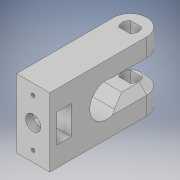
# Autodesk Inventor part: joint_2_part1
Saved by Autodesk Inventor 2019 (Build 230136000, 136)
## iProperties
Created: 2019-12-26
Part Number: joint_2_part1
Material: Типовые
Document SubType Name: Modeling
Designer: Петров Иван
Density: 1 g/cm^3
Appearance: По умолчанию
Author: Петров Иван
Autodesk Inventor part; units mm, degrees
ref_plane "YZ Plane" through (0, 0, 0) normal (1, 0, 0) x (0, 1, 0)
ref_plane "XZ Plane" through (0, 0, 0) normal (0, 1, 0) x (-1, 0, 0)
ref_plane "XY Plane" through (0, 0, 0) normal (0, 0, 1) x (1, 0, 0)
sketch "Эскиз1" plane through (0, 0, 0) normal (0, 1, 0) x (-1, 0, 0)
  arc A0 (6.0208, -6) -> (6.0208, 6) centre (0, 0) ccw
  line L0 (6.0208, -6) -> (-6.0208, -6)
  arc A1 (-6.0208, 6) -> (-6.0208, -6) centre (0, 0) ccw
  line L1 (6.0208, 6) -> (-6.0208, 6)
  line L2 (17.5, 37) -> (-17.5, 37)
  line L3 (-17.5, 37) -> (-17.5, 0)
  arc A2 (-17.5, 0) -> (17.5, 0) centre (0, 0) ccw
  line L4 (17.5, 0) -> (17.5, 37)
  line L5 (17.5, 0) -> (17.5, 57)
  line L6 (-17.5, 37) -> (17.5, 37)
  line L7 (17.5, 37) -> (17.5, 57)
  line L8 (17.5, 57) -> (-17.5, 57)
  line L9 (-17.5, 57) -> (-17.5, 37)
  constraints: 20 end point, 6 point on circle, 3 centre point, 2 parallel, 1 horizontal, 1 perpendicular
extrude "Выдавливание1" add sketch "Эскиз1" along normal blind 27
sketch "Эскиз2" plane through (-17.5, 0, 57) normal (0, 0, 1) x (1, 0, 0)
  line L0 (0, 0) -> (35, 0)
  line L1 (35, 0) -> (35, 72.2)
  line L2 (35, 72.2) -> (0, 72.2)
  line L3 (0, 72.2) -> (0, 0)
  point P0 (17.5, 0)
  dimension "d2" = 72.2
  constraints: 8 end point, 2 parallel, 1 horizontal, 1 perpendicular
  measures "d2" distance of L1.end L0.end
extrude "Выдавливание2" add sketch "Эскиз2" along normal blind 27
ref_plane "РабПлоскость1" through (17.5, 36.1, 84) normal (0, 1, 0) x (1, 0, 0)
mirror "Зеркальное отражение1" about plane through (17.5, 36.1, 84) normal (0, 1, 0) of "Выдавливание1"
sketch "Эскиз3" plane through (17.5, 0, 0) normal (1, 0, 0) x (0, 0, -1)
  line L0 (-57, 45.2) -> (-57, 27) projected
  line L1 (-57, 36.1) -> (-42, 36.1)
  circle A0 centre (-42, 36.1) radius 18
  point P0 (0, 0)
  dimension "d5" = 15
  dimension "d6" = 36
  constraints: 2 end point, 1 centre point, 1 coincident, 1 horizontal, 1 midpoint
  measures "d5" distance of L1.start L1.end
  measures "d6" diameter of A0
extrude "Выдавливание3" cut sketch "Эскиз3" against normal blind 93.5
chamfer "Фаска2" distance 8 angle 45 8 edges at (0, 27, 26.4697) (0, 45.2, 26.4697) (-17.5, 27, 13.2349) (0, 27, -17.5) (17.5, 27, 13.2349) (-17.5, 45.2, 13.2349) (0, 45.2, -17.5) (17.5, 45.2, 13.2349)
move faces "Перенос1" translate (0, 0, 18) faces at (-5.8333, 48.1333, 84)
sketch "Эскиз4" plane through (17.5, 36.1, 42) normal (1, 0, 0) x (0, 0, -1)
  line L0 (-60, -36.1) -> (-60, 36.1) projected
  line L1 (-60, 0) -> (-45, 0)
  line L2 (-52.5, -15) -> (-37.5, -15)
  line L3 (-37.5, -15) -> (-37.5, 15)
  line L4 (-37.5, 15) -> (-52.5, 15)
  line L5 (-52.5, 15) -> (-52.5, -15)
  line L6 (-52.5, -15) -> (-37.5, 15) construction
  line L7 (-37.5, -15) -> (-52.5, 15) construction
  point P0 (42, -36.1)
  dimension "d18" = 15
  dimension "d19" = 15
  dimension "d20" = 30
  constraints: 14 end point, 3 midpoint, 2 horizontal, 2 parallel, 1 perpendicular
  measures "d18" distance of L1.start L1.end
  measures "d19" distance of L4.end L3.end
  measures "d20" distance of L3.end L2.end
extrude "Выдавливание4" cut sketch "Эскиз4" against normal blind 79.25
sketch "Эскиз5" plane through (-17.5, 0, 102) normal (0, 0, 1) x (1, 0, 0)
  line L0 (23.5208, 72.2) -> (11.4792, 72.2) projected
  line L1 (17.5, 72.2) -> (17.5, 36.1)
  circle A0 centre (17.5, 36.1) radius 8
  point P0 (17.5, 0)
  dimension "d23" = 36.1
  dimension "d24" = 16
  constraints: 2 end point, 1 centre point, 1 coincident, 1 midpoint, 1 vertical
  measures "d23" distance of L1.start L1.end
  measures "d24" diameter of A0
extrude "Выдавливание5" cut sketch "Эскиз5" against normal blind 12.5
sketch "Эскиз14" plane through (-17.5, 0, 102) normal (0, 0, 1) x (1, 0, 0)
  circle A0 centre (17.5, 36.1) radius 8 projected
  line L0 (17.5, 36.1) -> (17.5, 61.1)
  circle A1 centre (17.5, 61.1) radius 1.9
  line L1 (17.5, 36.1) -> (17.5, 11.1)
  circle A2 centre (17.5, 11.1) radius 1.9
  point P0 (17.5, 0)
  dimension "d47" = 25
  dimension "d48" = 3.8
  dimension "d49" = 25
  dimension "d50" = 3.8
  constraints: 4 end point, 2 centre point, 2 coincident, 2 vertical
  measures "d47" distance of L0.start L0.end
  measures "d48" diameter of A1
  measures "d49" distance of L0.start L1.end
  measures "d50" diameter of A2
extrude "Выдавливание13" cut sketch "Эскиз14" against normal blind 20.35 contours A1 | A2
sketch "Эскиз15" plane through (-17.5, 0, 102) normal (0, 0, 1) x (1, 0, 0)
  circle A0 centre (17.5, 61.1) radius 1.9 projected
  circle A1 centre (17.5, 11.1) radius 1.9 projected
  circle A2 centre (17.5, 36.1) radius 8 projected
  line L0 (0, 0) -> (35, 0) projected
  line L1 (35, 0) -> (35, 72.2) projected
  line L2 (35, 72.2) -> (0, 72.2) projected
  line L3 (0, 72.2) -> (0, 0) projected
  point P0 (17.5, 0)
